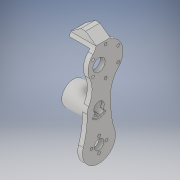
# Autodesk Inventor part: Frame_DC
Saved by Autodesk Inventor 2019 (Build 230136000, 136)
## iProperties
Created: 2019-07-29
Part Number: Frame_DC
Material: Generic
Document SubType Name: Modeling
Designer: 19879326
Density: 1 g/cm^3
Appearance: Default
Author: 19879326
Autodesk Inventor part; units mm, degrees
ref_plane "YZ Plane" through (0, 0, 0) normal (1, 0, 0) x (0, 1, 0)
ref_plane "XZ Plane" through (0, 0, 0) normal (0, 1, 0) x (-1, 0, 0)
ref_plane "XY Plane" through (0, 0, 0) normal (0, 0, 1) x (1, 0, 0)
sketch "Sketch1" plane through (0, 0, 0) normal (1, 0, 0) x (0, 1, 0)
  circle A0 centre (7, 0) radius 6.5
  circle A1 centre (-32, 0) radius 5.5
  circle A2 centre (-66.15, 0) radius 5.15
  arc A3 (-60.7004, 16.6299) -> (-60.7004, -16.6299) centre (-66.15, 0) ccw
  circle A4 centre (-58.15, 0) radius 1.5
  circle A5 centre (-66.15, 8) radius 1.5
  circle A6 centre (-74.15, 0) radius 1.5
  circle A7 centre (-66.15, -8) radius 1.5
  circle A8 centre (-32, 0) radius 12.5
  arc A9 (-60.7004, 16.6299) -> (-32.3393, 12.4954) centre (-34.6135, 96.2365) ccw
  arc A10 (25.953, -1.3181) -> (24.8491, 6.4234) centre (7.5, 0) ccw
  circle A11 centre (22.5, -7) radius 1.5
  circle A12 centre (-8.5, -7) radius 1.5
  circle A13 centre (14.75, 6.4234) radius 1.5
  circle A14 centre (-0.75, 6.4234) radius 1.5
  circle A15 centre (14.75, -20.4234) radius 1.5
  circle A16 centre (-0.75, -20.4234) radius 1.5
  arc A17 (19.7304, 6.4234) -> (25.453, -8.3181) centre (7, -7) ccw
  line L0 (24.8491, 6.4234) -> (19.7304, 6.4234)
  arc A18 (-25.8535, 10.8844) -> (-0.7032, 9.82) centre (-12.2351, 35) ccw
  arc A19 (-32.3393, -12.4954) -> (-60.7004, -16.6299) centre (-34.6135, -96.2365) ccw
  line L1 (25.953, -1.3181) -> (25.453, -8.3181)
  arc A20 (-5.5261, -20.6142) -> (-31.4249, -12.5252) centre (-27.0428, -44) ccw
  arc A21 (13.4162, 7.1097) -> (0.5838, 7.1097) centre (7, -7) ccw
  arc A22 (22.4274, -5.5018) -> (16.0112, 5.6114) centre (7, -7) ccw
  arc A23 (16.0112, -19.6114) -> (22.4274, -8.4982) centre (7, -7) ccw
  arc A24 (0.5838, -21.1097) -> (13.4162, -21.1097) centre (7, -7) ccw
  arc A25 (-2.0112, 5.6114) -> (-8.4274, -5.5018) centre (7, -7) ccw
  arc A26 (-8.4274, -8.4982) -> (-2.0112, -19.6114) centre (7, -7) ccw
  arc A27 (-30.6006, -12.4214) -> (-25.8535, 10.8844) centre (-32, 0) ccw
  arc A28 (-0.7032, 9.82) -> (-5.5261, -20.6142) centre (7, -7) ccw
  point P0 (0, 0)
  point P1 (0, 0)
  point P2 (-3.8164, -18.1021)
  point P3 (7.5, -18.5)
  point P4 (7, -25.5)
  dimension "d6" = 13
  dimension "d15" = 39
  dimension "d16" = 34.15
  dimension "d17" = 11
  dimension "d18" = 10.3
  dimension "d19" = 35
  dimension "d20" = 3
  dimension "d22" = 8
  dimension "d23" = 8
  dimension "d24" = 8
  dimension "d25" = 8
  dimension "d84" = 25
  dimension "d88" = 18.5
  dimension "d105" = 7
  dimension "d107" = 7
  dimension "d108" = 3
  dimension "d109" = 3
  dimension "d110" = 15.5
  dimension "d111" = 15.5
  dimension "d112" = 3
  dimension "d113" = 37
  dimension "d114" = 35
  dimension "d115" = 83.772
  dimension "d116" = 83.772
  dimension "d117" = 44
  dimension "d118" = 13.4234
  dimension "d119" = 0.5
  dimension "d120" = 15.5
  constraints: 52 point on circle, 29 centre point, 12 equal radius, 11 tangent, 9 horizontal alignment, 5 vertical alignment, 4 end point, 3 coincident, 1 horizontal
  measures "d6" diameter of A0
  measures "d15" distance of A0.centre A1.centre
  measures "d16" distance of A2.centre A1.centre
  measures "d17" diameter of A1
  measures "d18" diameter of A2
  measures "d19" diameter of A3
  measures "d20" diameter of A4
  measures "d22" distance of A2.centre A4.centre
  measures "d23" distance of A6.centre A2.centre
  measures "d24" distance of A5.centre A2.centre
  measures "d25" distance of A7.centre A2.centre
  measures "d84" diameter of A8
  measures "d88" radius of A10
  measures "d105" distance of point (0, 0) A0.centre
  measures "d107" distance of A0.centre A21.centre
  measures "d108" diameter of A11
  measures "d109" diameter of A12
  measures "d110" distance of A11.centre A13.centre
  measures "d111" distance of A14.centre A13.centre
  measures "d112" diameter of A15
  measures "d113" diameter of A17
  measures "d114" vertical distance of A1.centre A18.centre
  measures "d115" radius of A9
  measures "d116" radius of A19
  measures "d117" vertical distance of A20.centre A1.centre
  measures "d118" distance from line of A11.centre L0
  measures "d119" distance of A0.centre A10.centre
  measures "d120" radius of A26
extrude "Extrusion1" add sketch "Sketch1" along normal blind 5 contours A9 A8 A19 A3 | A8 | A18 A17 A20 A8 | A17 L0 A10 L1 | A11 A23 A15 A24 A16 A26 A12 A25 A14 A21 A13 A22
sketch "Sketch3" plane through (0, 0, 0) normal (-1, 0, 0) x (0, 0, 1)
  circle A0 centre (0, -32) radius 7.6
  circle A1 centre (0, -32) radius 5.5 projected
  point P0 (0, 0)
  dimension "d31" = 15.2
  constraints: 1 centre point, 1 concentric
  measures "d31" diameter of A0
extrude "Extrusion2" cut sketch "Sketch3" against normal blind 2
sketch "Sketch4" plane through (0, 0, 0) normal (-1, 0, 0) x (0, 0, 1)
  arc A0 (-11.4564, -37) -> (-11.4564, -27) centre (0, -32) ccw
  circle A1 centre (0, -32) radius 7.6 projected
  line L0 (-20, -49.15) -> (-20, 0) projected
  line L1 (-20, -40) -> (-20, -24)
  circle A2 centre (0, -32) radius 12.5
  point P0 (0, 0)
  point P1 (-18.5, 0)
  point P2 (-20, -32)
  dimension "d34" = 25
  constraints: 2 centre point, 2 concentric, 2 end point, 2 point on circle, 1 coincident, 1 horizontal alignment, 1 midpoint, 2 other
  measures "d34" diameter of A0
extrude "Extrusion3" add sketch "Sketch4" along normal blind 22
sketch "Sketch6" plane through (-22, 0, 0) normal (-1, 0, 0) x (0, 0, 1)
  arc A0 (-1.3197, -39.4845) -> (1.3197, -39.4845) centre (0, -32) ccw
  circle A1 centre (0, -32) radius 7.6 projected
  arc A2 (-1.5802, -40.9618) -> (-1.3197, -39.4845) centre (-1.45, -40.2231) ccw
  arc A3 (1.3197, -39.4845) -> (1.5802, -40.9618) centre (1.45, -40.2231) ccw
  line L0 (0, -32) -> (0, -39.6)
  circle A4 centre (0, -32) radius 7.6 projected
  arc A5 (1.5802, -40.9618) -> (-1.5802, -40.9618) centre (0, -32) ccw
  arc A6 (-7.1418, -39.1418) -> (7.1418, -39.1418) centre (0, -32) ccw
  arc A7 (-6.4347, -38.4347) -> (-7.1418, -39.1418) centre (-6.7882, -38.7882) ccw
  arc A8 (7.1418, -39.1418) -> (6.4347, -38.4347) centre (6.7882, -38.7882) ccw
  point P0 (0, 0)
  dimension "d48" = 10
  dimension "d49" = 10
  dimension "d50" = 45
  dimension "d51" = 45
  dimension "d52" = 1.5
  dimension "d53" = 1
  constraints: 19 point on circle, 7 centre point, 7 tangent, 2 coincident, 2 concentric, 2 end point, 2 equal radius, 1 vertical
  measures "d52" diameter of A2
  measures "d53" diameter of A7
extrude "Extrusion5" cut sketch "Sketch6" against normal blind 28 contours A0 A3 A5 A8 A6 A7 A2
sketch "Sketch7" plane through (5, 0, 0) normal (1, 0, 0) x (0, 0, -1)
  arc A0 (-5.374, -37.374) -> (5.374, -37.374) centre (0, -32) ccw
  arc A1 (1.3197, -39.4845) -> (-1.3197, -39.4845) centre (0, -32) ccw projected
  arc A2 (-1.3197, -39.4845) -> (1.3197, -39.4845) centre (0, -32) ccw projected
  arc A3 (-5.0445, -36.521) -> (-5.374, -37.374) centre (-5.0205, -37.0205) ccw
  arc A4 (5.374, -37.374) -> (5.0445, -36.521) centre (5.0205, -37.0205) ccw
  arc A5 (7.1418, -39.1418) -> (6.4347, -38.4347) centre (6.7882, -38.7882) ccw projected
  arc A6 (-6.4347, -38.4347) -> (-7.1418, -39.1418) centre (-6.7882, -38.7882) ccw projected
  line L0 (0, -32) -> (0, -39.6)
  arc A7 (-1.3197, -39.4845) -> (1.3197, -39.4845) centre (0, -32) ccw projected
  arc A8 (-5.0445, -36.521) -> (-4.4375, -35.2493) centre (-5.083, -35.722) ccw
  arc A9 (4.4375, -35.2493) -> (5.0445, -36.521) centre (5.083, -35.722) ccw
  circle A10 centre (0, -32) radius 5.5 projected
  arc A11 (-4.4375, -35.2493) -> (4.4375, -35.2493) centre (0, -32) ccw
  point P0 (0, 0)
  dimension "d56" = 45
  dimension "d57" = 45
  dimension "d61" = 0.8
  constraints: 18 point on circle, 7 tangent, 6 centre point, 4 equal radius, 2 end point, 1 coincident, 1 concentric
  measures "d61" radius of A8
extrude "Extrusion6" cut sketch "Sketch7" against normal blind 5 contours A3 A8 A10 L0 A0 | A0 L0 A10 A9 A4
sketch "Sketch12" plane through (0, 0, 0) normal (0, 0, 1) x (1, 0, 0)
  line L0 (0, 26) -> (5, 26) projected
  line L1 (5, 26) -> (-6, 34)
  line L2 (-6, 34) -> (-11, 34)
  line L3 (-11, 34) -> (-22, 26)
  line L4 (-22, 26) -> (5, 26)
  line L5 (5, 25.953) -> (5, 26) projected
  point P0 (0, 0)
  point P1 (5, 7.5)
  dimension "d89" = 27
  dimension "d90" = 8
  dimension "d91" = 5
  constraints: 8 end point, 2 point on line, 1 collinear, 1 equal length, 1 parallel
  measures "d89" distance of L3.end L1.start
  measures "d90" distance between parallel lines of L2 L4
  measures "d91" distance of L1.end L2.end
extrude "Extrusion11" add sketch "Sketch12" against normal blind 12
sketch "Sketch13" plane through (5, 0, 0) normal (1, 0, 0) x (0, 0, -1)
  line L0 (0, 26) -> (12, 26) projected
  line L1 (0, 26) -> (12, 26)
  line L2 (12, 26) -> (12, 21.5801)
  arc A0 (1.3181, 25.953) -> (0, 26) centre (0, 7.5) ccw projected
  arc A1 (12, 21.5801) -> (0, 26) centre (0, 7.5) ccw
  point P0 (0, 0)
  point P1 (18.5, 7.5)
  constraints: 4 end point, 3 point on circle, 1 centre point, 1 collinear, 1 concentric, 1 perpendicular
extrude "Extrusion12" add sketch "Sketch13" against normal blind 5
sketch "Sketch14" plane through (0, 0, 0) normal (0, 0, 1) x (1, 0, 0)
  line L0 (5, 26) -> (-6, 34) projected
  line L1 (-6, 34) -> (-11, 34) projected
  line L2 (-11, 34) -> (-22, 26) projected
  line L3 (-22, 26) -> (0, 26) projected
  line L4 (0, 26) -> (5, 26) projected
  point P0 (0, 0)
extrude "Extrusion13" add sketch "Sketch14" along normal blind 3
sketch "Sketch15" plane through (5, 0, 0) normal (1, 0, 0) x (0, 0, -1)
  line L0 (0, 26) -> (12, 26) projected
  line L1 (12, 26) -> (-3, 26) projected
  line L2 (0, 26) -> (-3, 26)
  line L3 (-3, 26) -> (-3, 25.7551)
  arc A0 (0, 26) -> (-6.4234, 24.8491) centre (0, 7.5) ccw projected
  arc A1 (0, 26) -> (-3, 25.7551) centre (0, 7.5) ccw
  point P0 (0, 0)
  point P1 (-18.5, 7.5)
  constraints: 4 end point, 3 point on circle, 1 centre point, 1 concentric, 1 horizontal, 1 perpendicular
extrude "Extrusion14" add sketch "Sketch15" against normal blind 5
sketch "Sketch16" plane through (0, 0, 0) normal (-1, 0, 0) x (0, 0, 1)
  line L0 (3, 26) -> (3, 25.7551) projected
  line L1 (6.4234, 24.8491) -> (6.4234, 19.7304) projected
  arc A0 (3, 25.7551) -> (6.4234, 19.7304) centre (16.9061, 29.6718) ccw
  arc A1 (9.82, -0.7032) -> (6.4234, 19.7304) centre (-7, 7) ccw projected
  arc A2 (6.4234, 24.8491) -> (3, 25.7551) centre (0, 7.5) ccw projected
  line L2 (6.4234, 24.8491) -> (6.4234, 19.7304) projected
  point P0 (0, 0)
  constraints: 2 point on circle, 1 centre point, 1 tangent
extrude "Extrusion15" cut sketch "Sketch16" against normal blind 10
sketch "Sketch17" plane through (0, 0, 0) normal (-1, 0, 0) x (0, 0, 1)
  arc A0 (4.6665, 21.9964) -> (-12, 25.3303) centre (-7, 7) ccw
  line L0 (-12, 24.8115) -> (-12, 26) projected
  line L1 (-12, 26) -> (-12, 25.4058)
  line L2 (-12, 26) -> (3, 26) projected
  line L3 (-12, 26) -> (-7, 26)
  line L4 (-7, 26) -> (3, 26)
  arc A1 (3, 25.7551) -> (6.4234, 19.7304) centre (16.9061, 29.6718) ccw projected
  line L5 (3, 26) -> (3, 25.7551)
  dimension "d123" = 38
  constraints: 8 end point, 4 point on circle, 2 point on line, 1 centre point, 1 coincident, 1 horizontal, 1 midpoint, 1 vertical
  measures "d123" diameter of A0
extrude "Extrusion16" add sketch "Sketch17" along normal blind 22
fillet "Fillet13" radius 2 1 edges at (2.5, 24.8115, -12)
body "Solid1"
